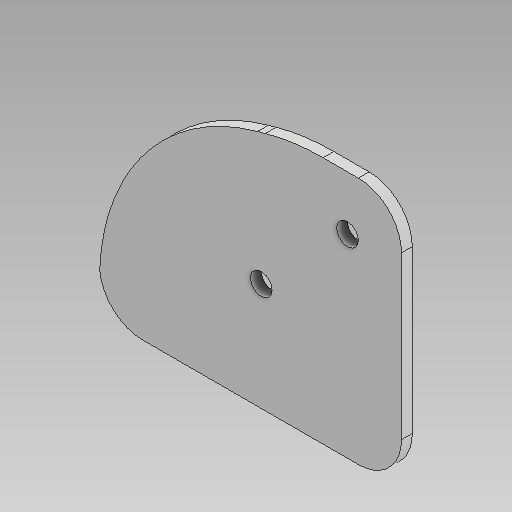
# Autodesk Inventor part: base
Saved by Autodesk Inventor 2025 (Build 290162000, 162)
## iProperties
Created: 2024-09-22
Part Number: base
Material: 일반
Document SubType Name: Modeling
Designer: OSB
Density: 1 g/cm^3
Appearance: 기본값
Author: OSB
Autodesk Inventor part; units mm, degrees
ref_plane "YZ Plane" through (0, 0, 0) normal (1, 0, 0) x (0, 1, 0)
ref_plane "XZ Plane" through (0, 0, 0) normal (0, 1, 0) x (-1, 0, 0)
ref_plane "XY Plane" through (0, 0, 0) normal (0, 0, 1) x (1, 0, 0)
sketch "스케치1" plane through (0, 0, 0) normal (0, 0, 1) x (1, 0, 0)
  circle A0 centre (0, 0) radius 5
  circle A1 centre (40, 40) radius 5
  line L0 (-55, -50) -> (45, -50)
  line L1 (65, -30) -> (65, 45)
  line L2 (45, 65) -> (28.6308, 65)
  line L3 (-75, -36.0086) -> (-75, -30)
  arc A2 (45, -50) -> (65, -30) centre (45, -30) ccw
  arc A3 (-75, -30) -> (-55, -50) centre (-55, -30) ccw
  arc A4 (65, 45) -> (45, 65) centre (45, 45) ccw
  line L4 (-1.7644, 60.3432) -> (1.8664, 61.3518)
  arc A5 (-1.7644, 60.3432) -> (-75, -36.0086) centre (25, -36.0086) ccw
  arc A6 (28.6308, 65) -> (1.8664, 61.3518) centre (28.6308, -35) ccw
  point P0 (-75, -50)
  point P1 (65, 65)
  point P2 (65, -50)
  point P3 (-75, 65)
  point P4 (-75, 40)
  point P5 (15, 65)
  point P6 (-74.9137, -31.8556)
  dimension "d0" = 10
  dimension "d1" = 10
  dimension "d2" = 40
  dimension "d3" = 40
  dimension "d4" = 75
  dimension "d5" = 50
  dimension "d6" = 25
  dimension "d7" = 25
  dimension "d10" = 20
  dimension "d11" = 25
  dimension "d12" = 25
  dimension "d13" = 100
  constraints: 12 point on line, 10 end point, 10 point on circle, 10 tangent, 7 centre point, 2 equal radius, 2 parallel, 1 coincident, 1 horizontal, 1 perpendicular
  measures "d0" diameter of A0
  measures "d1" diameter of A1
  measures "d2" horizontal distance of point (0, 0) A1.centre
  measures "d3" horizontal distance of point (0, 0) A1.centre
  measures "d4" distance from line of L3 point (0, 0)
  measures "d5" distance from line of L0 point (0, 0)
  measures "d6" distance from line of L1 A1.centre
  measures "d7" distance from line of L2 A1.centre
  measures "d10" radius of A2
  measures "d11" horizontal distance of point (15, 65) A1.centre
  measures "d12" distance from line of point (-75, 40) L2
  measures "d13" radius of A5
extrude "돌출1" add sketch "스케치1" along normal blind 5 contours A3 A5 L4 A6 L2 A4 L1 A2 L0
